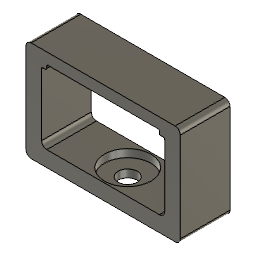
powerBoard (Autodesk Fusion 360 design; units mm, degrees)
part number: 2026-08-10-19-56-16-923
Autodesk Fusion 360 part; units mm, degrees
sketch "Sketch1" plane through (0, 0, 0) normal (0, 0, 1) x (1, 0, 0)
  line L0 (-28, 37) -> (62, 37)
  line L1 (62, 37) -> (62, 18)
  line L2 (62, 18) -> (-28, 18)
  line L3 (-28, 18) -> (-28, 37)
  dimension "d1" = 90
  dimension "d2" = 19
  constraint horizontal L0
  constraint vertical L1
  constraint horizontal L2
  constraint vertical L3
  measures "d1" distance of L0.start L0.end
  measures "d2" distance of L0.start L2.end
extrude "Extrude1" add sketch "Sketch1" along normal blind 6
sketch "Sketch2" plane through (0, 0, 6) normal (0, 0, 1) x (-1, 0, 0)
  line L0 (28, -37) -> (28, -18)
  line L1 (28, -18) -> (-62, -18)
  line L2 (-62, -18) -> (-62, -37)
  line L3 (-62, -37) -> (28, -37)
ref_plane "WorkPlane1" through (17, 27.5, 6) normal (0, 0, 1) x (-1, 0, 0)
sketch "Sketch3" plane through (0, 0, 6) normal (0, 0, 1) x (1, 0, 0)
  line L0 (17, 37) -> (17, 18)
  circle A0 centre (-8, 27.5) radius 8.9
  circle A1 centre (42, 27.5) radius 8.9
  circle A2 centre (-8, 27.5) radius 3.65
  circle A3 centre (42, 27.5) radius 3.65
  dimension "d13" = 17.8
  dimension "d14" = 17.8
  dimension "d15" = 7.3
  dimension "d16" = 7.3
  constraint vertical L0
  constraint concentric A0 A2
  constraint concentric A1 A3
  measures "d13" diameter of A0
  measures "d14" diameter of A1
  measures "d15" diameter of A2
  measures "d16" diameter of A3
extrude "Extrude2" cut sketch "Sketch3" against normal blind 7 contours A2 | A3
extrude "Extrude3" cut sketch "Sketch3" against normal blind 3
delete_face "DeleteFace1" 1 faces at (49.1033, 26.8765, 3)
ref_plane "WorkPlane3" through (17, 27.5, 6) normal (0, 0, 1) x (1, 0, 0)
sketch "Sketch7" plane through (0, 0, 6) normal (0, 0, 1) x (1, 0, 0)
  line L0 (-7.8773, 27.4561) -> (15.6227, 27.4561)
  line L1 (15.6227, 27.4561) -> (15.6227, 18)
  line L2 (15.6227, 18) -> (62, 18)
  line L3 (62, 18) -> (62, 37)
  line L4 (62, 37) -> (15.6227, 37)
  line L5 (15.6227, 37) -> (15.6227, 18)
  dimension "d38" = 23.5
  constraint horizontal L0
  constraint perpendicular L0 L1
  constraint horizontal L2
  constraint vertical L3
  constraint horizontal L4
  constraint vertical L5
  measures "d38" distance of L0.start L0.end
extrude "Extrude7" cut sketch "Sketch7" against normal blind 10
sketch "Sketch8" plane through (0, 0, 6) normal (0, 0, 1) x (-1, 0, 0)
  line L0 (-15.6227, -18) -> (-15.6227, -37)
  line L1 (-15.6227, -37) -> (28, -37)
  line L2 (28, -37) -> (28, -18)
  line L3 (28, -18) -> (-15.6227, -18)
  circle A0 centre (8, -27.5) radius 8.9
  line L4 (28, -37) -> (31.375, -37)
  line L5 (31.375, -37) -> (31.375, -18)
  line L6 (31.375, -18) -> (28, -18)
  line L7 (28, -18) -> (28, -37)
  dimension "d41" = 3.375
  dimension "d42" = 19
  constraint horizontal L4
  constraint vertical L5
  constraint horizontal L6
  constraint vertical L7
  constraint coincident L1.end L2.start
  measures "d41" distance of L1.end L4.end
  measures "d42" distance of L1.end L2.end
extrude "Extrude8" add sketch "Sketch8" against normal blind 6 contours L2 L4 L5 L6 L7
ref_plane "WorkPlane4" through (-7.8762, 18, 3) normal (0, -1, 0) x (1, 0, 0)
sketch "Sketch9" plane through (0, 18, 0) normal (0, -1, 0) x (-1, 0, 0)
  line L0 (-15.6, 0) -> (-21.6, 0)
  line L1 (-21.6, 0) -> (-21.6, -32.3)
  line L2 (-21.6, -32.3) -> (-15.6, -32.3)
  line L3 (-15.6, -32.3) -> (-15.6, 0)
  dimension "d46" = 6
  dimension "d47" = 32.3
  constraint horizontal L0
  constraint vertical L1
  constraint horizontal L2
  constraint vertical L3
  measures "d46" distance of L0.start L0.end
  measures "d47" distance of L0.start L2.end
extrude "Extrude9" add sketch "Sketch9" against normal blind 19
sketch "Sketch10" plane through (0, 37, 0) normal (0, 1, 0) x (-1, 0, 0)
  line L0 (-21.6, 0) -> (31.375, 0)
  line L1 (31.375, 0) -> (31.375, 6)
  line L2 (31.375, 6) -> (-15.6, 6)
  line L3 (-15.6, 6) -> (-15.6, 32.3)
  line L4 (-15.6, 32.3) -> (-21.6, 32.3)
  line L5 (-21.6, 32.3) -> (-21.6, 0)
  line L6 (31.375, 0) -> (37.375, 0)
  line L7 (37.375, 0) -> (37.375, 32.3)
  line L8 (37.375, 32.3) -> (31.375, 32.3)
  line L9 (31.375, 32.3) -> (31.375, 0)
  dimension "d50" = 6
  dimension "d51" = 32.3
  constraint horizontal L6
  constraint vertical L7
  constraint horizontal L8
  constraint vertical L9
  constraint coincident L0.end L1.start
  measures "d50" distance of L0.end L6.end
  measures "d51" distance of L0.end L8.end
extrude "Extrude10" add sketch "Sketch10" against normal blind 19 contours L1 L6 L7 L8 L9
sketch "Sketch11" plane through (0, 37, 0) normal (0, 1, 0) x (-1, 0, 0)
  line L0 (-21.6, 0) -> (37.375, 0)
  line L1 (37.375, 0) -> (37.375, 32.3)
  line L2 (37.375, 32.3) -> (31.375, 32.3)
  line L3 (31.375, 32.3) -> (31.375, 6)
  line L4 (31.375, 6) -> (-15.6, 6)
  line L5 (-15.6, 6) -> (-15.6, 32.3)
  line L6 (-15.6, 32.3) -> (-21.6, 32.3)
  line L7 (-21.6, 32.3) -> (-21.6, 0)
  line L8 (-21.6, 32.3) -> (37.375, 32.3)
  line L9 (37.375, 32.3) -> (37.375, 38.3)
  line L10 (37.375, 38.3) -> (-21.6, 38.3)
  line L11 (-21.6, 38.3) -> (-21.6, 32.3)
  dimension "d54" = 6
  constraint horizontal L8
  constraint vertical L9
  constraint horizontal L10
  constraint vertical L11
  constraint coincident L6.end L7.start
  measures "d54" distance of L6.end L10.end
extrude "Extrude11" add sketch "Sketch11" against normal blind 19 contours L2 L6 L8 L9 L10 L11
sketch "Sketch12" plane through (0, 37, 0) normal (0, 1, 0) x (-1, 0, 0)
  line L0 (31.375, 32.3) -> (31.375, 6)
  line L1 (31.375, 6) -> (-15.6, 6)
  line L2 (-15.6, 6) -> (-15.6, 32.3)
  line L3 (-15.6, 32.3) -> (31.375, 32.3)
  line L4 (37.375, 0) -> (37.375, 38.3)
  line L5 (37.375, 38.3) -> (-21.6, 38.3)
  line L6 (-21.6, 38.3) -> (-21.6, 0)
  line L7 (-21.6, 0) -> (37.375, 0)
  line L8 (-15.6, 32.3) -> (-13.6, 32.3)
  line L9 (31.375, 32.3) -> (29.375, 32.3)
  line L10 (-13.6, 32.3) -> (29.375, 32.3)
  line L11 (29.375, 32.3) -> (29.375, 34.0809)
  line L12 (29.375, 34.0809) -> (-13.6, 34.0809)
  line L13 (-13.6, 34.0809) -> (-13.6, 32.3)
  dimension "d57" = 2
  dimension "d58" = 2
  constraint coincident L2.end L3.start
  constraint perpendicular L2 L8
  constraint coincident L0.start L3.end
  constraint perpendicular L0 L9
  constraint horizontal L10
  constraint vertical L11
  constraint horizontal L12
  constraint vertical L13
  measures "d57" distance of L2.end L8.end
  measures "d58" distance of L0.start L9.end
extrude "Extrude12" cut sketch "Sketch12" against normal blind 19 contours L3 L10 L11 L12 L13
fillet "Fillet3" radius 2 3 edges at (-31.375, 27.5, 6) (21.6, 27.5, 38.3) (-37.375, 27.5, 38.3)
fillet "Fillet4" radius 2 2 edges at (15.6, 27.5, 6) (-37.375, 27.5, 0)
fillet "Fillet5" radius 2 1 edges at (21.6, 27.5, 0)
fillet "Fillet6" radius 0.5 1 edges at (-29.375, 27.5, 32.3)
fillet "Fillet7" radius 0.5 3 edges at (-31.375, 27.5, 32.3) (-29.375, 27.5, 34.0809) (13.6, 27.5, 32.3)
fillet "Fillet8" radius 0.5 2 edges at (15.6, 27.5, 32.3) (13.6, 27.5, 34.0809)
